Autodesk Inventor part; units mm, degrees
(part 2 of 2)
sketch "Sketch3" plane through (0, 0, -1.6) normal (0, 0, -1) x (-1, 0, 0)
  line L0 (118.8796, -36.2425) -> (-0.1826, -42.8058) projected
  line L1 (-0.1826, 42.8058) -> (118.8796, 36.2425) projected
  line L2 (-0.1826, -3.175) -> (-0.1826, -36.2777) projected
  line L3 (-4.8972, -43.0657) -> (-129.6442, -49.9424) projected
  line L4 (-129.6442, 49.9424) -> (-4.8972, 43.0657) projected
  line L5 (-4.8972, -36.5376) -> (-4.8972, -3.175) projected
  line L6 (-0.1826, -76.5762) -> (-0.1826, -42.8058) projected
  line L7 (-0.1826, -66.4337) -> (-4.8972, -66.4337)
  line L8 (-4.8972, -77.1018) -> (-4.8972, -43.0657) projected
  line L9 (-4.8972, -53.7337) -> (-0.1826, -53.7337)
  line L10 (-4.8972, -26.2063) -> (-0.1826, -26.2063)
  line L11 (-4.8972, -13.5063) -> (-0.1826, -13.5063)
  line L12 (-0.1826, -36.2777) -> (-0.1826, -3.175) projected
  line L13 (-4.8972, 3.175) -> (-4.8972, 36.5376) projected
  line L14 (-4.8972, 13.5063) -> (-0.1826, 13.5063)
  line L15 (-0.1826, 36.2777) -> (-0.1826, 3.175) projected
  line L16 (-0.1826, 26.2063) -> (-5.1182, 26.2063)
  line L17 (-5.044, 53.7337) -> (-0.1826, 53.7337)
  line L18 (-0.1826, 42.8058) -> (-0.1826, 76.5762) projected
  line L19 (-0.1826, 66.4337) -> (-4.8972, 66.4337)
  line L20 (-4.8972, 77.1018) -> (-4.8972, 43.0657) projected
  line L21 (122.0546, -56.1227) -> (115.7046, -56.1227)
  line L22 (115.7046, -56.1227) -> (115.7046, -43.4227)
  line L23 (115.7046, -43.4227) -> (122.0546, -43.4227)
  line L24 (122.0546, -43.4227) -> (122.0546, -56.1227)
  line L25 (118.8796, -63.3029) -> (118.8796, -36.2425) projected
  line L26 (122.0546, -56.1227) -> (115.7046, -43.4227) construction
  line L27 (115.7046, -56.1227) -> (122.0546, -43.4227) construction
  line L28 (122.0546, -22.7947) -> (115.7046, -22.7947)
  line L29 (115.7046, -22.7947) -> (115.7046, -10.0947)
  line L30 (115.7046, -10.0947) -> (122.0546, -10.0947)
  line L31 (122.0546, -10.0947) -> (122.0546, -22.7947)
  line L32 (118.8796, -3.175) -> (118.8796, -29.7144) projected
  line L33 (122.0546, -22.7947) -> (115.7046, -10.0947) construction
  line L34 (115.7046, -22.7947) -> (122.0546, -10.0947) construction
  line L35 (122.0546, 10.0947) -> (115.7046, 10.0947)
  line L36 (115.7046, 10.0947) -> (115.7046, 22.7947)
  line L37 (115.7046, 22.7947) -> (122.0546, 22.7947)
  line L38 (122.0546, 22.7947) -> (122.0546, 10.0947)
  line L39 (118.8796, 29.7144) -> (118.8796, 3.175) projected
  line L40 (122.0546, 10.0947) -> (115.7046, 22.7947) construction
  line L41 (115.7046, 10.0947) -> (122.0546, 22.7947) construction
  line L42 (122.0546, 43.4227) -> (115.7046, 43.4227)
  line L43 (115.7046, 43.4227) -> (115.7046, 56.1227)
  line L44 (115.7046, 56.1227) -> (122.0546, 56.1227)
  line L45 (122.0546, 56.1227) -> (122.0546, 43.4227)
  line L46 (118.8796, 36.2425) -> (118.8796, 63.3029) projected
  line L47 (122.0546, 43.4227) -> (115.7046, 56.1227) construction
  line L48 (115.7046, 43.4227) -> (122.0546, 56.1227) construction
  line L49 (-126.4692, -80.0006) -> (-132.8192, -80.0006)
  line L50 (-132.8192, -80.0006) -> (-132.8192, -60.9506)
  line L51 (-132.8192, -60.9506) -> (-126.4692, -60.9506)
  line L52 (-126.4692, -60.9506) -> (-126.4692, -80.0006)
  line L53 (-129.6442, -49.9424) -> (-129.6442, -91.0088) projected
  line L54 (-126.4692, -80.0006) -> (-132.8192, -60.9506) construction
  line L55 (-132.8192, -80.0006) -> (-126.4692, -60.9506) construction
  line L56 (-126.4692, -32.8196) -> (-132.8192, -32.8196)
  line L57 (-132.8192, -32.8196) -> (-132.8192, -13.7696)
  line L58 (-132.8192, -13.7696) -> (-126.4692, -13.7696)
  line L59 (-126.4692, -13.7696) -> (-126.4692, -32.8196)
  line L60 (-129.6442, -43.4142) -> (-129.6442, -3.175) projected
  line L61 (-126.4692, -32.8196) -> (-132.8192, -13.7696) construction
  line L62 (-132.8192, -32.8196) -> (-126.4692, -13.7696) construction
  line L63 (-126.4692, 13.7696) -> (-132.8192, 13.7696)
  line L64 (-132.8192, 13.7696) -> (-132.8192, 32.8196)
  line L65 (-132.8192, 32.8196) -> (-126.4692, 32.8196)
  line L66 (-126.4692, 32.8196) -> (-126.4692, 13.7696)
  line L67 (-129.6442, 3.175) -> (-129.6442, 43.4142) projected
  line L68 (-126.4692, 13.7696) -> (-132.8192, 32.8196) construction
  line L69 (-132.8192, 13.7696) -> (-126.4692, 32.8196) construction
  line L70 (-126.4692, 60.9506) -> (-132.8192, 60.9506)
  line L71 (-132.8192, 60.9506) -> (-132.8192, 80.0006)
  line L72 (-132.8192, 80.0006) -> (-126.4692, 80.0006)
  line L73 (-126.4692, 80.0006) -> (-126.4692, 60.9506)
  line L74 (-129.6442, 91.0088) -> (-129.6442, 49.9424) projected
  line L75 (-126.4692, 60.9506) -> (-132.8192, 80.0006) construction
  line L76 (-132.8192, 60.9506) -> (-126.4692, 80.0006) construction
  line L77 (-4.8972, 77.1018) -> (-129.6442, 91.0088) construction
  line L78 (-129.6442, -91.0088) -> (-4.8972, -77.1018) construction
  line L79 (0, 0) -> (118.8796, 0) construction
  line L80 (118.8796, 0) -> (59.4398, 0)
  line L81 (59.4398, 0) -> (0, 0)
  line L82 (0, 0) -> (29.7199, 0)
  line L83 (29.7199, 0) -> (59.4398, 0)
  line L84 (59.4398, 0) -> (89.1597, 0)
  line L85 (89.1597, 0) -> (118.8796, 0)
  line L86 (108.4646, 82.0683) -> (99.5746, 82.0683)
  line L87 (99.5746, 82.0683) -> (99.5746, -82.0683)
  line L88 (99.5746, -82.0683) -> (108.4646, -82.0683)
  line L89 (108.4646, -82.0683) -> (108.4646, 82.0683)
  line L90 (108.4646, 82.0683) -> (99.5746, -82.0683) construction
  line L91 (99.5746, 82.0683) -> (108.4646, -82.0683) construction
  line L92 (78.7447, 86.2449) -> (69.8547, 86.2449)
  line L93 (69.8547, 86.2449) -> (69.8547, -86.2449)
  line L94 (69.8547, -86.2449) -> (78.7447, -86.2449)
  line L95 (78.7447, -86.2449) -> (78.7447, 86.2449)
  line L96 (78.7447, 86.2449) -> (69.8547, -86.2449) construction
  line L97 (69.8547, 86.2449) -> (78.7447, -86.2449) construction
  line L98 (-0.1826, -97.3369) -> (118.8796, -80.6046) projected
  line L99 (49.0248, 90.4216) -> (40.1348, 90.4216)
  line L100 (40.1348, 90.4216) -> (40.1348, -90.4216)
  line L101 (40.1348, -90.4216) -> (49.0248, -90.4216)
  line L102 (49.0248, -90.4216) -> (49.0248, 90.4216)
  line L103 (49.0248, 90.4216) -> (40.1348, -90.4216) construction
  line L104 (40.1348, 90.4216) -> (49.0248, -90.4216) construction
  line L105 (19.3049, 94.5982) -> (10.4149, 94.5982)
  line L106 (10.4149, 94.5982) -> (10.4149, -94.5982)
  line L107 (10.4149, -94.5982) -> (19.3049, -94.5982)
  line L108 (19.3049, -94.5982) -> (19.3049, 94.5982)
  line L109 (19.3049, 94.5982) -> (10.4149, -94.5982) construction
  line L110 (10.4149, 94.5982) -> (19.3049, -94.5982) construction
  line L111 (-4.8972, 0) -> (-129.6442, 0) construction
  line L112 (-4.8972, -3.175) -> (-129.6442, -3.175) construction
  line L113 (0, 0) -> (-4.8972, 0) construction
  line L114 (-4.8972, 0) -> (-67.2707, 0) construction
  line L115 (-67.2707, 0) -> (-129.6442, 0) construction
  line L116 (-129.6442, 0) -> (-98.4575, 0) construction
  line L117 (-67.2707, 0) -> (-98.4575, 0) construction
  line L118 (-67.2707, 0) -> (-36.084, 0) construction
  line L119 (-36.084, 0) -> (-4.8972, 0) construction
  line L120 (-16.0456, 99.5662) -> (-24.9356, 99.5662)
  line L121 (-24.9356, 99.5662) -> (-24.9356, -99.5662)
  line L122 (-24.9356, -99.5662) -> (-16.0456, -99.5662)
  line L123 (-16.0456, -99.5662) -> (-16.0456, 99.5662)
  line L124 (-16.0456, 99.5662) -> (-24.9356, -99.5662) construction
  line L125 (-24.9356, 99.5662) -> (-16.0456, -99.5662) construction
  line L126 (-47.2324, 103.949) -> (-56.1224, 103.949)
  line L127 (-56.1224, 103.949) -> (-56.1224, -103.949)
  line L128 (-56.1224, -103.949) -> (-47.2324, -103.949)
  line L129 (-47.2324, -103.949) -> (-47.2324, 103.949)
  line L130 (-47.2324, 103.949) -> (-56.1224, -103.949) construction
  line L131 (-56.1224, 103.949) -> (-47.2324, -103.949) construction
  line L132 (-78.4191, 108.3318) -> (-87.3091, 108.3318)
  line L133 (-87.3091, 108.3318) -> (-87.3091, -108.3318)
  line L134 (-87.3091, -108.3318) -> (-78.4191, -108.3318)
  line L135 (-78.4191, -108.3318) -> (-78.4191, 108.3318)
  line L136 (-78.4191, 108.3318) -> (-87.3091, -108.3318) construction
  line L137 (-87.3091, 108.3318) -> (-78.4191, -108.3318) construction
  line L138 (-118.4959, 112.7146) -> (-109.6059, 112.7146)
  line L139 (-109.6059, 112.7146) -> (-109.6059, -112.7146)
  line L140 (-109.6059, -112.7146) -> (-118.4959, -112.7146)
  line L141 (-118.4959, -112.7146) -> (-118.4959, 112.7146)
  line L142 (-118.4959, 112.7146) -> (-109.6059, -112.7146) construction
  line L143 (-109.6059, 112.7146) -> (-118.4959, -112.7146) construction
  line L144 (-129.6442, -115.5306) -> (-4.8972, -97.9994) projected
  point P0 (-68.3972, -46.5662)
  point P1 (-4.8972, -60.0837)
  point P2 (-4.8972, -19.8563)
  point P3 (-4.8972, 19.8563)
  point P4 (-4.8972, 60.0837)
  point P5 (-4.8972, 53.7337)
  point P6 (-4.8972, 26.2063)
  point P7 (-0.1826, -13.5063)
  point P8 (118.8796, -49.7727)
  point P9 (118.8796, -16.4447)
  point P10 (118.8796, 16.4447)
  point P11 (118.8796, 49.7727)
  point P12 (-129.6442, -70.4756)
  point P13 (-129.6442, -23.2946)
  point P14 (-129.6442, 23.2946)
  point P15 (-129.6442, 70.4756)
  point P16 (-129.6442, 32.8196)
  point P17 (-129.6442, 13.7696)
  point P18 (104.0196, 0)
  point P19 (74.2997, 0)
  point P20 (44.5798, 0)
  point P21 (14.8599, 0)
  point P22 (-20.4906, 0)
  point P23 (-51.6774, 0)
  point P24 (-82.8641, 0)
  point P25 (-114.0509, 0)
  dimension "d8" = 12.7
  dimension "d9" = 6.35
  dimension "d10" = 12.7
  dimension "d11" = 6.35
  dimension "d12" = 12.7
  dimension "d13" = 6.35
  dimension "d14" = 12.7
  dimension "d15" = 6.35
  dimension "d18" = 6.35
  dimension "d19" = 12.7
  dimension "d20" = 6.35
  dimension "d21" = 12.7
  dimension "d22" = 6.35
  dimension "d23" = 12.7
  dimension "d24" = 6.35
  dimension "d25" = 12.7
  dimension "d26" = 6.35
  dimension "d27" = 19.05
  dimension "d28" = 6.35
  dimension "d29" = 19.05
  dimension "d30" = 6.35
  dimension "d31" = 19.05
  dimension "d32" = 6.35
  dimension "d33" = 19.05
  dimension "d34" = 8.89
  dimension "d35" = 8.89
  dimension "d36" = 8.89
  dimension "d37" = 8.89
  dimension "d38" = 8.89
  dimension "d39" = 8.89
  dimension "d40" = 8.89
  dimension "d41" = 8.89
  constraints: 238 end point, 57 midpoint, 37 parallel, 24 point on line, 20 perpendicular, 17 horizontal, 7 collinear, 3 other
  measures "d8" distance between parallel lines of L7 L9
  measures "d9" distance from line of L7 point (-4.897, -60.084)
  measures "d10" distance between parallel lines of L10 L11
  measures "d11" distance from line of point (-4.897, -19.856) L11
  measures "d12" distance between parallel lines of L14 L16
  measures "d13" distance from line of point (-4.897, 19.856) L16
  measures "d14" distance between parallel lines of L17 L19
  measures "d15" distance from line of point (-4.897, 60.084) L19
  measures "d18" distance of L22.end L23.end
  measures "d19" distance of L21.end L22.end
  measures "d20" distance of L29.end L30.end
  measures "d21" distance of L28.end L29.end
  measures "d22" distance of L36.end L37.end
  measures "d23" distance of L35.end L36.end
  measures "d24" distance of L43.end L44.end
  measures "d25" distance of L42.end L43.end
  measures "d26" distance of L50.end L51.end
  measures "d27" distance of L49.end L50.end
  measures "d28" distance of L57.end L58.end
  measures "d29" distance of L56.end L57.end
  measures "d30" distance of L64.end L65.end
  measures "d31" distance of L63.end L64.end
  measures "d32" distance of L71.end L72.end
  measures "d33" distance of L70.end L71.end
  measures "d34" distance of L88.end L87.end
  measures "d35" distance of L94.end L93.end
  measures "d36" distance of L101.end L100.end
  measures "d37" distance of L107.end L106.end
  measures "d38" distance of L122.end L121.end
  measures "d39" distance of L128.end L127.end
  measures "d40" distance of L134.end L133.end
  measures "d41" distance of L139.end L140.end
extrude "Extrusion3" add sketch "Sketch3" against normal blind 1.6 contours L51 L52 L49 L53 | L53 L49 L50 L51 | L70 L71 L72 L74 | L74 L72 L73 L70 | L42 L43 L44 L46 | L46 L44 L45 L42 | L89 L88 L87 L0 | L0 L87 L80 L89 | L23 L24 L21 L25 | L25 L21 L22 L23 | L80 L87 L1 L89 | L95 L94 L93 L0 | L0 L93 L80 L95 | L1 L87 L86 L89 | L80 L93 L1 L95 | L101 L100 L0 L102 | L0 L100 L81 L102 | L1 L93 L92 L95 | L107 L106 L0 L108 | L81 L100 L1 L102 | L0 L106 L81 L108 | L1 L100 L99 L102 | L81 L106 L1 L108 | L1 L106 L105 L108 | L6 L7 L8 L9 | L17 L20 L19 L18 | L123 L122 L121 L3 | L3 L121 L4 L123 | L4 L121 L120 L123 | L129 L128 L127 L3 | L3 L127 L4 L129 | L4 L127 L126 L129 | L134 L133 L3 L135 | L3 L133 L4 L135 | L140 L141 L3 L139 | L4 L133 L132 L135 | L3 L141 L4 L139 | L4 L141 L138 L139 | L2 L10 L5 L11 | L13 L16 L15 L14 | L28 L32 L30 L31 | L28 L29 L30 L32 | L35 L39 L37 L38 | L35 L36 L37 L39 | L56 L60 L58 L59 | L56 L57 L58 L60 | L63 L67 L65 L66 | L63 L64 L65 L67
equation "\"d9\" = 0.5 * d8"
equation "\"d11\" = 0.5 * d10"
equation "\"d13\" = 0.5 * d12"
equation "\"d15\" = 0.5 * d14"
body "Solid1"
